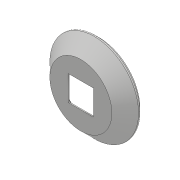
# Autodesk Inventor part: sensor_holder
Saved by Autodesk Inventor 2017 (Build 210142000, 142)
## iProperties
Created: 2018-10-30
Part Number: sensor_holder
Material: Generic
Document SubType Name: Modeling
Designer: mfans
Density: 1 g/cm^3
Appearance: Default
Author: mfans
Autodesk Inventor part; units mm, degrees
ref_plane "YZ Plane" through (0, 0, 0) normal (1, 0, 0) x (0, 1, 0)
ref_plane "XZ Plane" through (0, 0, 0) normal (0, 1, 0) x (-1, 0, 0)
ref_plane "XY Plane" through (0, 0, 0) normal (0, 0, 1) x (1, 0, 0)
sketch "Sketch1" plane through (0, 0, 0) normal (0, 0, 1) x (1, 0, 0)
  line L0 (0, 0) -> (30.9497, 0)
  line L1 (30.9497, 0) -> (44.9497, 14)
  line L2 (0, 0) -> (0, 14)
  line L3 (44.9497, 14) -> (40, 18.9497)
  line L4 (0, 14) -> (40, 14)
  line L5 (40, 14) -> (40, 18.9497)
  dimension "d1" = 45
  dimension "d2" = 14
  dimension "d3" = 90
  dimension "d4" = 7
  dimension "d5" = 40
  constraints: 12 end point, 2 horizontal, 1 perpendicular, 1 vertical
  measures "d1" angle of L0 L1
  measures "d2" distance of L0.start L2.end
  measures "d3" angle of L1 L3
  measures "d4" distance of L1.end L3.end
  measures "d5" distance between parallel lines of L2 L5
revolve "Revolution1" add sketch "Sketch1" angle 360 about axis through (0, 0, 0) along (0, 1, 0)
shell "Shell1" thickness 1 removed faces 2 at (-36.8857, 17.2998, -15.474) at (-6.0893, 14, -16.5433)
fillet "Fillet1" radius 0.5 1 edges at (-40, 18.9497, 0)
sketch "Sketch2" plane through (0, 0, 0) normal (0, 0, 1) x (1, 0, 0)
  line L0 (40.8536, 18.0962) -> (44.9497, 14) projected
  point P0 (0, 0)
surface extrude "ExtrusionSrf1" sketch "Sketch2" along normal mid plane 20 shown no curves L0
sketch "Sketch3" plane through (44.9497, 14, -10) normal (0.7071068, 0.7071068, 0) x (-0.7071068, 0.7071068, 0)
  line L0 (0.6464, 8.6479) -> (0.6464, 11.3521)
  line L1 (5.1464, 8.6479) -> (5.1464, 11.3521)
  arc A0 (0.6464, 8.6479) -> (5.1464, 8.6479) centre (2.8964, 10) ccw
  arc A1 (5.1464, 11.3521) -> (0.6464, 11.3521) centre (2.8964, 10) ccw
  line L2 (2.8964, 10) -> (0, 10)
  line L3 (0, 10) -> (2.8964, 10)
  ellipse E0 centre (34.6807, 10) end of major axis (34.6807, 50.8536) minor radius 28.8878 projected
  line L4 (5.7929, 10) -> (2.8964, 10)
  line L5 (0, 0) -> (0, 20) projected
  point P0 (21.8848, 10)
  dimension "d12" = 4.5
  constraints: 10 end point, 4 equal length, 4 point on circle, 2 centre point, 2 horizontal, 1 horizontal alignment, 1 midpoint, 1 point on line, 1 vertical, 1 other
  measures "d12" distance between parallel lines of L0 L1
extrude "Extrusion1" cut sketch "Sketch3" against normal blind 0.5 contours L0 L2 L4 L1 A0 | L0 A1 L1 L4 L2
sketch "Sketch4" plane through (44.5962, 13.6464, -10) normal (0.7071068, 0.7071068, 0) x (0, 0, 1)
  circle A0 centre (10, -2.8964) radius 2.6238
  arc A1 (11.3521, -5.1464) -> (11.3521, -0.6464) centre (10, -2.8964) ccw projected
  point P0 (10, -21.8848)
  point P1 (11.75, -2.8964)
  point P2 (8.25, -2.8964)
  dimension "d15" = 1.75
  dimension "d16" = 1.75
  constraints: 2 vertical alignment, 1 centre point, 1 concentric
  measures "d15" distance of point (11.75, -2.896) A0.centre
  measures "d16" distance of A0.centre point (8.25, -2.896)
hole "Hole1" at (42.5481, 15.6945, 1.75) at (42.5481, 15.6945, -1.75) direction (-0.7071068, -0.7071068, 0) diameter 1 end up to face face through (-7.6187, 1, -6.7496) facing (0, 1, 0)
pattern_circular "Circular Pattern1" count 4 over 360 about axis through (0, -10, 0) along (0, 1, 0) of "Extrusion1", "Hole1"
fillet "Fillet2" radius 1 1 edges at (-44.9497, 14, 0)
fillet "Fillet3" radius 2 1 edges at (-43.5355, 14, 0)
sketch "Sketch5" plane through (0, 1, 0) normal (0, 1, 0) x (1, 0, 0)
  line L0 (12.5, -12.5) -> (-12.5, -12.5)
  line L1 (-12.5, -12.5) -> (-12.5, 12.5)
  line L2 (-12.5, 12.5) -> (12.5, 12.5)
  line L3 (12.5, 12.5) -> (12.5, -12.5)
  line L4 (12.5, -12.5) -> (-12.5, 12.5) construction
  line L5 (-12.5, -12.5) -> (12.5, 12.5) construction
  point P0 (0, 0)
  dimension "d29" = 25
  dimension "d30" = 25
  constraints: 12 end point, 2 midpoint, 2 parallel, 1 horizontal, 1 perpendicular
  measures "d29" distance between parallel lines of L0 L2
  measures "d30" distance of L1.end L2.end
extrude "Extrusion2" cut sketch "Sketch5" against normal blind 10
body "Solid1"
body "Srf1"
